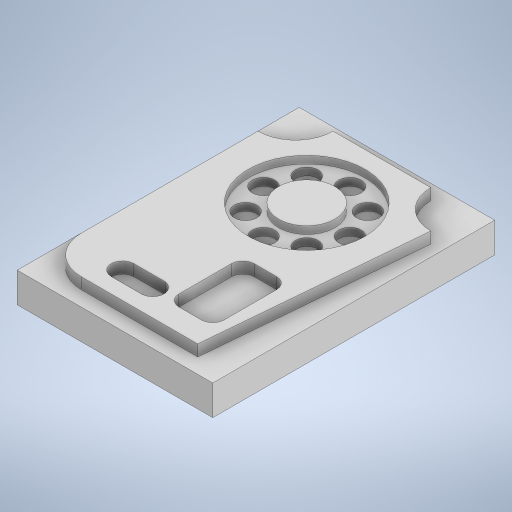
# Autodesk Inventor part: Exercise2
Saved by Autodesk Inventor 2023 (Build 270158000, 158)
## iProperties
Created: 2023-04-25
Part Number: Exercise2
Material: Generic
Document SubType Name: Modeling
Designer: dell
Density: 1 g/cm^3
Appearance: Default
Author: dell
Autodesk Inventor part; units mm, degrees
ref_plane "YZ Plane" through (0, 0, 0) normal (1, 0, 0) x (0, 1, 0)
ref_plane "XZ Plane" through (0, 0, 0) normal (0, 1, 0) x (-1, 0, 0)
ref_plane "XY Plane" through (0, 0, 0) normal (0, 0, 1) x (1, 0, 0)
sketch "Sketch1" plane through (0, 0, 0) normal (0, 1, 0) x (-1, 0, 0)
  line L0 (26, 37.5) -> (-26, 37.5)
  line L1 (-26, 37.5) -> (-26, -37.5)
  line L2 (-26, -37.5) -> (26, -37.5)
  line L3 (26, -37.5) -> (26, 37.5)
  line L4 (26, 37.5) -> (-26, -37.5) construction
  line L5 (-26, 37.5) -> (26, -37.5) construction
  point P0 (0, 0)
  dimension "d0" = 52
  dimension "d1" = 75
  constraints: 12 end point, 2 midpoint, 2 parallel, 1 horizontal, 1 perpendicular
  measures "d0" distance of L1.end L2.end
  measures "d1" distance of L2.end L0.start
extrude "Extrusion1" add sketch "Sketch1" along normal blind 8
sketch "Sketch2" plane through (0, 8, 0) normal (0, 1, 0) x (1, 0, 0)
  arc A0 (-23, 23.5) -> (-13, 33.5) centre (-23, 33.5) ccw
  line L0 (26, 37.5) -> (-26, 37.5) projected
  line L1 (-26, 37.5) -> (-26, -37.5) projected
  arc A1 (13, 33.5) -> (23, 23.5) centre (23, 33.5) ccw
  line L2 (26, -37.5) -> (26, 37.5) projected
  line L3 (-13, 33.5) -> (13, 33.5)
  line L4 (-23, -23.5) -> (-23, 27.9055)
  arc A2 (-23, -23.5) -> (-13, -33.5) centre (-13, -23.5) ccw
  line L5 (-13, -33.5) -> (18, -33.5)
  line L6 (-26, -37.5) -> (26, -37.5) projected
  line L7 (18, -33.5) -> (23, 23.5)
  line L8 (7, -27.5) -> (13, -27.5)
  line L9 (16, -24.5) -> (16, -10.5)
  line L10 (13, -7.5) -> (7, -7.5)
  line L11 (4, -10.5) -> (4, -24.5)
  line L12 (4, -27.5) -> (16, -7.5) construction
  line L13 (16, -27.5) -> (4, -7.5) construction
  line L14 (-9, -29.5) -> (-0.6728, -29.5)
  line L15 (-0.6728, -23.5) -> (-9, -23.5)
  line L16 (-9, -29.5) -> (-0.6728, -23.5) construction
  line L17 (-0.6728, -29.5) -> (-9, -23.5) construction
  arc A3 (-9, -23.5) -> (-9, -29.5) centre (-9, -26.5) ccw
  arc A4 (-0.6728, -29.5) -> (-0.6728, -23.5) centre (-1, -26.5) ccw
  arc A5 (4, -24.5) -> (7, -27.5) centre (7, -24.5) ccw
  arc A6 (7, -7.5) -> (4, -10.5) centre (7, -10.5) ccw
  arc A7 (16, -10.5) -> (13, -7.5) centre (13, -10.5) ccw
  arc A8 (13, -27.5) -> (16, -24.5) centre (13, -24.5) ccw
  point P0 (0, 0)
  point P1 (10, -17.5)
  point P2 (-4.8364, -26.5)
  dimension "d4" = 20
  dimension "d5" = 4
  dimension "d6" = 3
  dimension "d7" = 4
  dimension "d8" = 3
  dimension "d9" = 20
  dimension "d10" = 3
  dimension "d14" = 3
  dimension "d15" = 4
  dimension "d18" = 8
  dimension "d19" = 16
  dimension "d20" = 22
  dimension "d22" = 4
  dimension "d23" = 20
  dimension "d24" = 30
  dimension "d25" = 10
  dimension "d26" = 6
  dimension "d27" = 6
  dimension "d29" = 11
  dimension "d30" = 27
  dimension "d31" = 35
  dimension "d32" = 49
  dimension "d33" = 52
  dimension "d38" = 3
  constraints: 28 end point, 18 point on circle, 10 tangent, 9 centre point, 4 midpoint, 3 parallel, 3 perpendicular, 2 horizontal, 1 point on line, 1 vertical
  measures "d4" diameter of A0
  measures "d5" distance from line of L0 A0.centre
  measures "d6" distance from line of L1 A0.centre
  measures "d7" distance from line of L0 A1.centre
  measures "d8" distance from line of L2 A1.centre
  measures "d9" diameter of A1
  measures "d10" distance between parallel lines of L4 L1
  measures "d14" distance from line of L7.end L2
  measures "d15" distance between parallel lines of L0 L3
  measures "d18" distance from line of L2 L5.end
  measures "d19" distance from line of L2 point (10, -17.5)
  measures "d20" distance between parallel lines of L2 L11
  measures "d22" distance from line of L6 L5.end
  measures "d23" distance from line of L6 point (10, -17.5)
  measures "d24" distance between parallel lines of L6 L10
  measures "d25" radius of A2
  measures "d26" distance between parallel lines of L14 L15
  measures "d27" diameter of A3
  measures "d29" distance from line of L6 A4.centre
  measures "d30" distance from line of L2 A4.centre
  measures "d31" distance from line of L2 A3.centre
  measures "d32" distance between parallel lines of L2 L4
  measures "d33" distance between parallel lines of L2 L1
  measures "d38" radius of A7
extrude "Extrusion2" add sketch "Sketch2" along normal blind 3 contours A0 L3 A1 L7 L5 A2 L4
sketch "Sketch3" plane through (0, 11, 0) normal (0, 1, 0) x (1, 0, 0)
  circle A0 centre (0, 13.5) radius 15.5
  circle A1 centre (0, 13.5) radius 7.5
  line L0 (-26, -37.5) -> (26, -37.5) projected
  line L1 (26, -37.5) -> (26, 37.5) projected
  point P0 (0, 0)
  dimension "d41" = 15
  dimension "d42" = 31
  dimension "d43" = 51
  dimension "d44" = 26
  constraints: 2 centre point, 1 coincident
  measures "d41" diameter of A1
  measures "d42" diameter of A0
  measures "d43" distance from line of L0 A0.centre
  measures "d44" distance from line of L1 A0.centre
extrude "Extrusion3" cut sketch "Sketch3" against normal blind 2
sketch "Sketch4" plane through (0, 9, -13.5) normal (0, 1, 0) x (1, 0, 0)
  circle A0 centre (0, 0) radius 7.5 projected
  circle A1 centre (0, 0) radius 11.5
  circle A2 centre (11.5, 0) radius 3
  circle A3 centre (8.1317, 8.1317) radius 3
  circle A4 centre (0, 11.5) radius 3
  circle A5 centre (-8.1317, 8.1317) radius 3
  circle A6 centre (-11.5, 0) radius 3
  circle A7 centre (-8.1317, -8.1317) radius 3
  circle A8 centre (0, -11.5) radius 3
  circle A9 centre (8.1317, -8.1317) radius 3
  point P0 (0, -13.5)
  dimension "d47" = 23
  dimension "d48" = 6
  dimension "d51" = 360
  constraints: 8 centre point, 1 coincident, 1 horizontal alignment, 19 other
  measures "d48" diameter of A2
extrude "Extrusion4" cut sketch "Sketch4" against normal blind 2 contours A1 A2 | A1 A2 | A3 A1 | A1 A3 | A9 A1 | A1 A9 | A4 A1 | A1 A4 | A8 A1 | A1 A8 | A5 A1 | A1 A5 | A7 A1 | A1 A7 | A6 A1 | A1 A6
body "Solid1"
